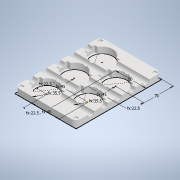
# Autodesk Inventor part: trayTop
Saved by Autodesk Inventor 2022 (Build 260153000, 153)
## iProperties
Created: 2023-05-08
Part Number: trayTop
Material: Generic
Document SubType Name: Modeling
Designer: Hallgato
Density: 1 g/cm^3
Appearance: Default
Author: Hallgato
Autodesk Inventor part; units mm, degrees
ref_plane "YZ Plane" through (0, 0, 0) normal (1, 0, 0) x (0, 1, 0)
ref_plane "XZ Plane" through (0, 0, 0) normal (0, 1, 0) x (-1, 0, 0)
ref_plane "XY Plane" through (0, 0, 0) normal (0, 0, 1) x (1, 0, 0)
sketch "Sketch1" plane through (0, 0, 0) normal (0, 1, 0) x (-1, 0, 0)
  circle A0 centre (0, 0) radius 17.75
  line L0 (0, 0) -> (0, -10.9961) construction
  circle A1 centre (0, -45) radius 17.75
  circle A2 centre (45, 22.5) radius 17.75
  circle A3 centre (45, -22.5) radius 17.75
  circle A4 centre (45, -67.5) radius 17.75
  line L1 (-27.5, -92.5) -> (72.5, -92.5)
  line L2 (72.5, -92.5) -> (72.5, 47.5)
  line L3 (72.5, 47.5) -> (-27.5, 47.5)
  line L4 (-27.5, 47.5) -> (-27.5, -92.5)
  line L5 (-27.5, -92.5) -> (72.5, 47.5) construction
  line L6 (72.5, -92.5) -> (-27.5, 47.5) construction
  point P0 (22.5, -22.5)
  dimension "d0" = 35.5
  dimension "d3" = 45
  dimension "d8" = 35.5
  dimension "d9" = 45
  dimension "d10" = 22.5
  dimension "d13" = 45
  dimension "d18" = 22.5
  dimension "d19" = 50
  dimension "d20" = 70
  dimension "d21" = 22.5
  constraints: 14 end point, 5 centre point, 3 vertical, 2 midpoint, 2 parallel, 1 coincident, 1 horizontal, 1 perpendicular, 6 other
  measures "d0" diameter of A0
  measures "d3" distance of L0.start A1.centre
  measures "d8" diameter of A2
  measures "d9" horizontal distance of A2.centre point (0, 0)
  measures "d10" vertical distance of point (0, 0) A2.centre
  measures "d13" distance of A2.centre A3.centre
  measures "d18" distance of point (22.5, -22.5) A3.centre
  measures "d19" distance from line of L4 point (22.5, -22.5)
  measures "d20" distance from line of L1 point (22.5, -22.5)
  measures "d21" horizontal distance of point (22.5, -22.5) A1.centre
extrude "Extrusion1" add sketch "Sketch1" along normal blind 10
extrude "Extrusion2" add sketch "Sketch1" against normal blind 3 contours A0 | A1 | A2 | A3 | A4 | L4 L3 L2 L1
sketch "Sketch3" plane through (-72.5, 10, -92.5) normal (-1, 0, 0) x (0, 0, 1)
  ellipse E0 centre (25, 0) end of major axis (25, 4.95) minor radius 4.9499
  ellipse E1 centre (70, 0) end of major axis (70, 4.95) minor radius 4.9499
  ellipse E2 centre (115, 0) end of major axis (115, 4.95) minor radius 4.9499
  ellipse E3 centre (47.5, 0) end of major axis (47.5, 4.95) minor radius 4.95
  ellipse E4 centre (92.5, 0) end of major axis (92.5, 4.95) minor radius 4.9499
  line L0 (7.25, 0) -> (42.75, 0) construction
  line L1 (29.75, 0) -> (65.25, 0) projected
  point P0 (92.5, -10)
  dimension "d40" = 17.75
  dimension "d41" = 17.75
  dimension "d42" = 22.5
  dimension "d43" = 22.5
  dimension "d44" = 22.5
  constraints: 5 centre point
  measures "d40" distance of L0.start E0.centre
  measures "d41" distance of L1.start E3.centre
  measures "d42" distance of E1.centre E3.centre
  measures "d43" distance of E4.centre E1.centre
  measures "d44" distance of E4.centre E2.centre
extrude "Extrusion3" cut sketch "Sketch3" along normal mid plane 300
sketch "Sketch4" plane through (0, 10, 0) normal (0, 1, 0) x (1, 0, 0)
  line L0 (-62.0459, -27.4499) -> (-72.5, -27.4499) projected
  line L1 (-72.5, -17.5501) -> (-62.0459, -17.5501) projected
  line L2 (-62.0459, 17.5501) -> (-72.5, 17.5501) projected
  line L3 (-72.5, 27.4499) -> (-62.0459, 27.4499) projected
  line L4 (-62.0459, 62.5501) -> (-72.5, 62.5501) projected
  line L5 (-72.5, 72.4499) -> (-62.0459, 72.4499) projected
  line L6 (-65.5, -31.4499) -> (-57, -31.4499)
  line L7 (-57, -31.4499) -> (-57, -13.5501)
  line L8 (-57, -13.5501) -> (-65.5, -13.5501)
  line L9 (-65.5, -13.5501) -> (-65.5, -31.4499)
  line L10 (-72.5, 62.5501) -> (-72.5, 72.4499) projected
  line L11 (-72.5, 92.5) -> (-72.5, 72.4499) projected
  line L12 (-72.5, -47.5) -> (-72.5, 92.5) projected
  line L13 (-72.5, -27.4499) -> (-72.5, -47.5) projected
  line L14 (-72.5, -27.4499) -> (-72.5, -17.5501) projected
  line L15 (-72.5, -4.9499) -> (-72.5, -17.5501) projected
  line L16 (-72.5, 17.5501) -> (-72.5, 27.4499) projected
  line L17 (-72.5, 17.5501) -> (-72.5, 4.9499) projected
  line L18 (-72.5, -4.9499) -> (-72.5, 4.9499) projected
  line L19 (-72.5, 40.05) -> (-72.5, 27.4499) projected
  line L20 (-72.5, 40.05) -> (-72.5, 49.95) projected
  line L21 (-72.5, 62.5501) -> (-72.5, 49.95) projected
  line L22 (27.5, -4.9499) -> (17.0459, -4.9499) projected
  line L23 (27.5, 40.05) -> (17.0458, 40.05) projected
  line L24 (17.0459, 4.9499) -> (27.5, 4.9499) projected
  line L25 (17.0458, 49.95) -> (27.5, 49.95) projected
  line L26 (-17.0458, 40.05) -> (-42.3432, 40.05) projected
  line L27 (-42.3432, 49.95) -> (-17.0458, 49.95) projected
  line L28 (-27.9541, 27.4499) -> (27.5, 27.4499) projected
  line L29 (27.5, 17.5501) -> (2.6561, 17.5501) projected
  line L30 (-2.6561, 17.5501) -> (-27.9541, 17.5501) projected
  line L31 (-27.9541, -17.5501) -> (27.5, -17.5501) projected
  line L32 (27.5, -27.4499) -> (-27.9541, -27.4499) projected
  line L33 (-27.9541, 72.4499) -> (27.5, 72.4499) projected
  line L34 (27.5, 62.5501) -> (-27.9541, 62.5501) projected
  circle A0 centre (-45, -22.5) radius 17.75 projected
  circle A1 centre (-45, 22.5) radius 17.75 projected
  circle A2 centre (-45, 67.5) radius 17.75 projected
  circle A3 centre (0, 45) radius 17.75 projected
  circle A4 centre (0, 0) radius 17.75 projected
  line L35 (-45, -22.5) -> (-45, -14.8529) construction
  line L36 (-45, -22.5) -> (-37.3529, -22.5) construction
  line L37 (-24.5, -31.4499) -> (-33, -31.4499)
  line L38 (-33, -31.4499) -> (-33, -13.5501)
  line L39 (-33, -13.5501) -> (-24.5, -13.5501)
  line L40 (-24.5, -13.5501) -> (-24.5, -31.4499)
  line L41 (-65.5, 13.2698) -> (-57, 13.2698)
  line L42 (-57, 13.2698) -> (-57, 31.1695)
  line L43 (-57, 31.1695) -> (-65.5, 31.1695)
  line L44 (-65.5, 31.1695) -> (-65.5, 13.2698)
  line L45 (-24.5, 31.1695) -> (-24.5, 13.2698)
  line L46 (-24.5, 13.2698) -> (-33, 13.2698)
  line L47 (-33, 13.2698) -> (-33, 31.1695)
  line L48 (-33, 31.1695) -> (-24.5, 31.1695)
  line L49 (-65.5, 58.2698) -> (-57, 58.2698)
  line L50 (-57, 58.2698) -> (-57, 76.1695)
  line L51 (-57, 76.1695) -> (-65.5, 76.1695)
  line L52 (-65.5, 76.1695) -> (-65.5, 58.2698)
  line L53 (-24.5, 76.1695) -> (-24.5, 58.2698)
  line L54 (-24.5, 58.2698) -> (-33, 58.2698)
  line L55 (-33, 58.2698) -> (-33, 76.1695)
  line L56 (-33, 76.1695) -> (-24.5, 76.1695)
  line L57 (-20.5, 35.7698) -> (-12, 35.7698)
  line L58 (-12, 35.7698) -> (-12, 53.6695)
  line L59 (-12, 53.6695) -> (-20.5, 53.6695)
  line L60 (-20.5, 53.6695) -> (-20.5, 35.7698)
  line L61 (20.5, 53.6695) -> (20.5, 35.7698)
  line L62 (20.5, 35.7698) -> (12, 35.7698)
  line L63 (12, 35.7698) -> (12, 53.6695)
  line L64 (12, 53.6695) -> (20.5, 53.6695)
  line L65 (-20.5, -9.2302) -> (-12, -9.2302)
  line L66 (-12, -9.2302) -> (-12, 8.6695)
  line L67 (-12, 8.6695) -> (-20.5, 8.6695)
  line L68 (-20.5, 8.6695) -> (-20.5, -9.2302)
  line L69 (20.5, 8.6695) -> (20.5, -9.2302)
  line L70 (20.5, -9.2302) -> (12, -9.2302)
  line L71 (12, -9.2302) -> (12, 8.6695)
  line L72 (12, 8.6695) -> (20.5, 8.6695)
  point P0 (-65.5, -27.4499)
  point P1 (15.4888, 8.6695)
  point P2 (15.1614, -9.2302)
  point P3 (15.4888, 53.6695)
  point P4 (15.1614, 35.7698)
  dimension "d29" = 4
  dimension "d30" = 4
  dimension "d31" = 12
  dimension "d32" = 8.5
  dimension "d33" = 90
  dimension "d34" = 8.5
  dimension "d35" = 8.5
  dimension "d36" = 8.5
  dimension "d37" = 8.5
  constraints: 84 end point, 10 parallel, 6 horizontal, 6 perpendicular, 4 symmetric about line, 2 point on line
  measures "d29" distance between parallel lines of L8 L1
  measures "d30" distance between parallel lines of L6 L0
  measures "d31" distance from line of L7 L35.start
  measures "d32" distance between parallel lines of L9 L7
  measures "d33" angle of L36 L35
  measures "d34" distance between parallel lines of L44 L42
  measures "d35" distance between parallel lines of L52 L50
  measures "d36" distance between parallel lines of L60 L58
  measures "d37" distance between parallel lines of L68 L66
extrude "Extrusion4" cut sketch "Sketch4" against normal up to surface (10 mm away) contours A0 L6 L9 L0 | L0 L9 L1 A0 | A0 L8 L7 L6 | L1 L9 L8 A0 | L37 L38 L39 A0 | A0 L32 L40 L37 | L39 L40 L31 A0 | A0 L31 L40 L32 | L44 L3 A1 L2 | L2 A1 L41 L44 | L65 L68 L67 A4 | A4 L67 L66 L65 | A1 L43 L42 L41 | L44 L43 A1 L3 | A4 L22 L69 L70 | A4 L24 L69 L22 | L46 L47 L48 A1 | A1 L30 L45 L46 | L30 A1 L28 L45 | L52 L5 A2 L4 | L4 A2 L49 L52 | L24 A4 L72 L69 | L28 A1 L48 L45 | L60 L27 A3 L26 | L26 A3 L57 L60 | A2 L51 L50 L49 | L52 L51 A2 L5 | A3 L59 L58 L57 | L60 L59 A3 L27 | A3 L23 L61 L62 | L54 L55 L56 A2 | A2 L34 L53 L54 | L56 L53 L33 A2 | A3 L25 L61 L23 | A2 L33 L53 L34 | L25 A3 L64 L61
sketch "Sketch5" plane through (0, 10, 0) normal (0, 1, 0) x (1, 0, 0)
  line L0 (-69.5, -44.5) -> (-64.5, -44.5)
  line L1 (-64.5, -44.5) -> (-64.5, -39.5)
  line L2 (-64.5, -39.5) -> (-69.5, -39.5)
  line L3 (-69.5, -39.5) -> (-69.5, -44.5)
  line L4 (-72.5, -47.5) -> (27.5, -47.5) projected
  line L5 (-72.5, -27.4499) -> (-72.5, -47.5) projected
  line L6 (-69.5, 84.5) -> (-64.5, 84.5)
  line L7 (-64.5, 84.5) -> (-64.5, 89.5)
  line L8 (-64.5, 89.5) -> (-69.5, 89.5)
  line L9 (-69.5, 89.5) -> (-69.5, 84.5)
  line L10 (19.5, 84.5) -> (24.5, 84.5)
  line L11 (24.5, 84.5) -> (24.5, 89.5)
  line L12 (24.5, 89.5) -> (19.5, 89.5)
  line L13 (19.5, 89.5) -> (19.5, 84.5)
  line L14 (19.5, -44.5) -> (24.5, -44.5)
  line L15 (24.5, -44.5) -> (24.5, -39.5)
  line L16 (24.5, -39.5) -> (19.5, -39.5)
  line L17 (19.5, -39.5) -> (19.5, -44.5)
  line L18 (27.5, 92.5) -> (-72.5, 92.5) projected
  line L19 (27.5, -47.5) -> (27.5, -27.4499) projected
  point P0 (0, 0)
  dimension "d45" = 5
  dimension "d46" = 5
  dimension "d47" = 3
  dimension "d48" = 3
  dimension "d49" = 5
  dimension "d50" = 3
  dimension "d51" = 5
  dimension "d52" = 3
  constraints: 32 end point, 8 collinear, 8 parallel, 4 horizontal, 4 perpendicular
  measures "d45" distance of L2.end L1.end
  measures "d46" distance of L1.end L0.end
  measures "d47" distance between parallel lines of L4 L0
  measures "d48" distance between parallel lines of L5 L3
  measures "d49" distance between parallel lines of L8 L6
  measures "d50" distance between parallel lines of L18 L8
  measures "d51" distance between parallel lines of L17 L15
  measures "d52" distance between parallel lines of L19 L15
extrude "Extrusion5" cut sketch "Sketch5" against normal blind 2
fillet "Fillet1" radius 8 4 edges at (27.5, 3.5, -92.5) (27.5, 3.5, 47.5) (-72.5, 3.5, 47.5) (-72.5, 3.5, -92.5)
fillet "Fillet2" radius 4 8 edges at (25.1569, -3, -90.1569) (27.5, -3, -22.5) (25.1569, -3, 45.1569) (-22.5, -3, 47.5) (-70.1569, -3, 45.1569) (-72.5, -3, -22.5) (-70.1569, -3, -90.1569) (-22.5, -3, -92.5)
equation "\"d0\" = bottleCap"
equation "\"d3\" = bottleDistance"
equation "\"d8\" = bottleCap"
equation "\"d9\" = bottleDistance"
equation "\"d10\" = 0.5 * bottleDistance"
equation "\"d13\" = bottleDistance"
equation "\"d18\" = 0.5 * bottleDistance"
equation "\"d21\" = 0.5 * bottleDistance"
equation "\"d40\" = 0.5 * bottleCap"
equation "\"d41\" = 0.5 * bottleCap"
equation "\"capDiameter\" = 29.5"
equation "\"bottleLen\" = 81.3"
equation "\"bottleDiameter\" = 38.8"
equation "\"tubeInsideDiameter\" = 2"
equation "\"tubeOutsideDiameter\" = 5.4"
equation "\"tick\" = 2"
equation "\"connectorDiameter\" = 35"
equation "\"connectorInsideDiameter\" = tubeInsideDiameter - tick"
equation "\"connectorTubeDepth\" = 18.5"
equation "\"tubeFlapDepth\" = 3"
equation "\"tubeFlapAngle\" = 15deg"
equation "\"minTick\" = 0.25"
equation "\"tubeLinkTick\" = 2"
equation "\"tubeTolerance\" = 0.3"
equation "\"tickHolder\" = 1"
equation "\"bottleDistance\" = 45"
equation "\"bottleCap\" = 35.5"
body "Solid1"
